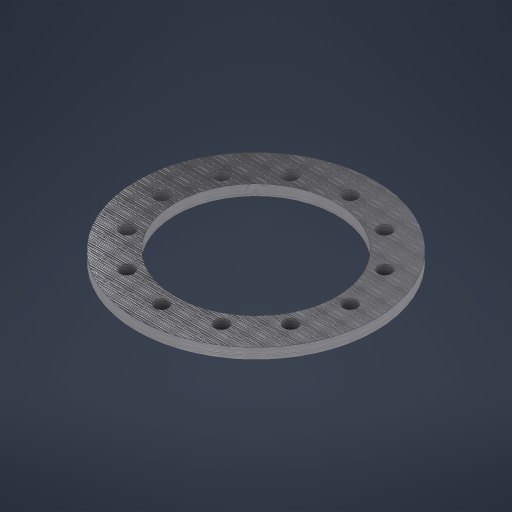
# Autodesk Inventor part: TurnTableSpacerPlate
Saved by Autodesk Inventor 2024 (Build 280153000, 153)
## iProperties
Created: 2023-10-25
Part Number: TurnTableSpacerPlate
Material: Generic
Document SubType Name: Modeling
Designer: avsar
Density: 1 g/cm^3
Appearance: Machined 03
Author: avsar
Autodesk Inventor part; units mm, degrees
ref_plane "YZ Plane" through (0, 0, 0) normal (1, 0, 0) x (0, 1, 0)
ref_plane "XZ Plane" through (0, 0, 0) normal (0, 1, 0) x (-1, 0, 0)
ref_plane "XY Plane" through (0, 0, 0) normal (0, 0, 1) x (1, 0, 0)
sketch "Sketch1" plane through (0, 0, 0) normal (0, 1, 0) x (-1, 0, 0)
  circle A0 centre (0, 0) radius 71
  circle A1 centre (0, 0) radius 48
  dimension "d0" = 142
  dimension "d1" = 96
  constraints: 2 centre point, 2 coincident
  measures "d0" diameter of A0
  measures "d1" diameter of A1
extrude "Extrusion1" add sketch "Sketch1" along normal blind 6.35
sketch "Sketch2" plane through (0, 6.35, 0) normal (0, 1, 0) x (1, 0, 0)
  circle A0 centre (0, 56) radius 4
  circle A1 centre (-28, 48.4974) radius 4
  circle A2 centre (-48.4974, 28) radius 4
  circle A3 centre (-56, 0) radius 4
  circle A4 centre (-48.4974, -28) radius 4
  circle A5 centre (-28, -48.4974) radius 4
  circle A6 centre (0, -56) radius 4
  circle A7 centre (28, -48.4974) radius 4
  circle A8 centre (48.4974, -28) radius 4
  circle A9 centre (56, 0) radius 4
  circle A10 centre (48.4974, 28) radius 4
  circle A11 centre (28, 48.4974) radius 4
  point P0 (0, 0)
  dimension "d4" = 8
  dimension "d5" = 56
  dimension "d8" = 360
  constraints: 12 centre point, 1 vertical alignment, 25 other
  measures "d4" diameter of A0
  measures "d5" distance of point (0, 0) A0.centre
extrude "Extrusion2" cut sketch "Sketch2" against normal through all
body "Solid1"
